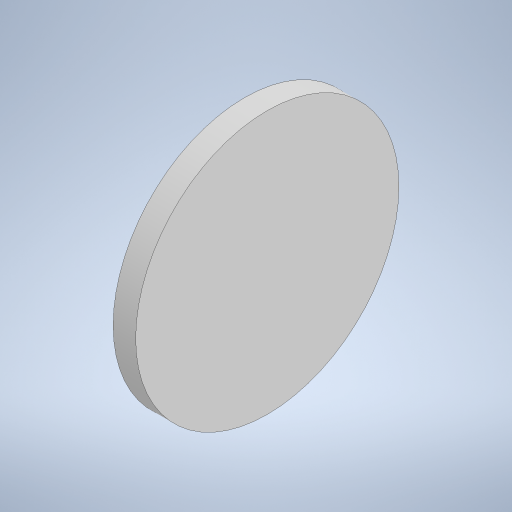
# Autodesk Inventor part: MAGNETPLATE CONCEPT
Saved by Autodesk Inventor 2023 (Build 270158000, 158)
## iProperties
Created: 2022-09-19
Part Number: MAGNETPLATE CONCEPT
Material: Generic
Document SubType Name: Modeling
Designer: D.C. Eksteen
Density: 1 g/cm^3
Appearance: Default
Author: D.C. Eksteen
Autodesk Inventor part; units mm, degrees
ref_plane "YZ Plane" through (0, 0, 0) normal (1, 0, 0) x (0, 1, 0)
ref_plane "XZ Plane" through (0, 0, 0) normal (0, 1, 0) x (-1, 0, 0)
ref_plane "XY Plane" through (0, 0, 0) normal (0, 0, 1) x (1, 0, 0)
sketch "Sketch1" plane through (0, 0, 0) normal (1, 0, 0) x (0, 1, 0)
  circle A0 centre (0, 0) radius 35
  dimension "d0" = 70
  constraints: 1 centre point, 1 coincident
  measures "d0" diameter of A0
extrude "Extrusion1" add sketch "Sketch1" along normal blind 5
sketch "Sketch2" plane through (5, 0, 0) normal (1, 0, 0) x (0, 0, -1)
  circle A0 centre (0, 0) radius 35 projected
  circle A1 centre (0, 0) radius 23 construction
  point P0 (23, 0)
  point P1 (16.2635, 16.2635)
  point P2 (0, 23)
  point P3 (-16.2635, 16.2635)
  point P4 (-23, 0)
  point P5 (-16.2635, -16.2635)
  point P6 (0, -23)
  point P7 (16.2635, -16.2635)
  dimension "d3" = 46
  dimension "d6" = 360
  constraints: 2 horizontal alignment, 1 coincident, 11 other
hole "Hole1" at (5, 0, -23) at (5, 16.2635, -16.2635) at (5, 23, 0) at (5, 16.2635, 16.2635) at (5, 0, 23) at (5, -16.2635, 16.2635) at (5, -23, 0) at (5, -16.2635, -16.2635) direction (-1, 0, 0) diameter 15 end through all
sketch "Sketch3" plane through (5, 0, 0) normal (1, 0, 0) x (0, 0, -1)
  circle A0 centre (0, -23) radius 7.5 projected
  circle A1 centre (-23, 0) radius 7.5 projected
  circle A2 centre (0, 23) radius 7.5 projected
  circle A3 centre (23, 0) radius 7.5 projected
  circle A4 centre (16.2635, 16.2635) radius 7.5 projected
  circle A5 centre (-16.2635, 16.2635) radius 7.5 projected
  circle A6 centre (-16.2635, -16.2635) radius 7.5 projected
  circle A7 centre (16.2635, -16.2635) radius 7.5 projected
  circle A8 centre (0, 0) radius 35 projected
extrude "Extrusion2" add sketch "Sketch3" along normal blind 1 contours A0 | A1 | A2 | A3 | A4 | A5 | A6 | A7 | A8
body "Solid1"
